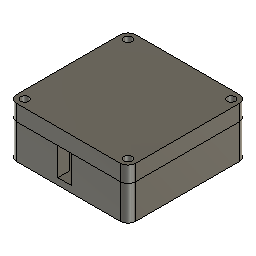
Wireless Charching Case (Autodesk Fusion 360 design; units mm, degrees)
Autodesk Fusion 360 part; units mm, degrees
sketch "Skizze1" plane through (0, 0, 0) normal (0, 0, 1) x (1, 0, 0)
  line L0 (15, -17.5) -> (-15, -17.5)
  line L1 (-17.5, -15) -> (-17.5, 15)
  line L2 (-15, 17.5) -> (15, 17.5)
  line L3 (17.5, 15) -> (17.5, -15)
  line L4 (17.5, -17.5) -> (-17.5, 17.5) construction
  line L5 (-17.5, -17.5) -> (17.5, 17.5) construction
  circle A0 centre (-15, 15) radius 1.5
  arc A1 (-15, 17.5) -> (-17.5, 15) centre (-15, 15) ccw
  arc A2 (-17.5, -15) -> (-15, -17.5) centre (-15, -15) ccw
  arc A3 (15, -17.5) -> (17.5, -15) centre (15, -15) ccw
  arc A4 (17.5, 15) -> (15, 17.5) centre (15, 15) ccw
  circle A5 centre (15, 15) radius 1.5
  circle A6 centre (-15, -15) radius 1.5
  circle A7 centre (15, -15) radius 1.5
  dimension "d1" = 35
  dimension "d2" = 35
  dimension "d3" = 3
  dimension "d4" = 2.5
  dimension "d5" = 2.5
  dimension "d8" = 30
  dimension "d9" = -30
  constraint horizontal L0
  constraint perpendicular L0 L1
  constraint parallel L0 L2
  constraint parallel L1 L3
  constraint coincident L4 origin
  constraint coincident L5 origin
  constraint coincident L4 A0.centre
  constraint coincident L4.end L2
  constraint coincident L4.end L1
  constraint tangent L2 A1
  constraint tangent L1 A1
  constraint coincident L5.start L1
  constraint coincident L5.start L0
  constraint tangent L1 A2
  constraint tangent L0 A2
  constraint equal A1 A2
  constraint coincident L4.start L0
  constraint coincident L4.start L3
  constraint tangent L0 A3
  constraint tangent L3 A3
  constraint equal A1 A3
  constraint coincident L5.end L3
  constraint coincident L5.end L2
  constraint tangent L3 A4
  constraint tangent L2 A4
  constraint equal A1 A4
  measures "d1" distance of L4.end L5.end
  measures "d2" distance of L5.start L4.end
  measures "d3" diameter of A0
  measures "d5" distance of L2 A0.centre
sketch "Skizze2" plane through (0, 0, 0) normal (0, 0, 1) x (1, 0, 0)
  line L0 (19.5, -22.5) -> (-19.5, -22.5)
  line L1 (-22.5, -19.5) -> (-22.5, 19.5)
  line L2 (-19.5, 22.5) -> (19.5, 22.5)
  line L3 (22.5, 19.5) -> (22.5, -19.5)
  line L4 (22.5, -22.5) -> (-22.5, 22.5) construction
  line L5 (-22.5, -22.5) -> (22.5, 22.5) construction
  arc A0 (-19.5, 22.5) -> (-22.5, 19.5) centre (-19.5, 19.5) ccw
  arc A1 (22.5, 19.5) -> (19.5, 22.5) centre (19.5, 19.5) ccw
  arc A2 (19.5, -22.5) -> (22.5, -19.5) centre (19.5, -19.5) ccw
  arc A3 (-22.5, -19.5) -> (-19.5, -22.5) centre (-19.5, -19.5) ccw
  line L6 (15, -18) -> (-15, -18)
  line L7 (-18, -15) -> (-18, 15)
  line L8 (-15, 18) -> (15, 18)
  line L9 (18, 15) -> (18, -15)
  line L10 (18, -18) -> (-18, 18) construction
  line L11 (-18, -18) -> (18, 18) construction
  arc A4 (-15, 18) -> (-18, 15) centre (-15, 15) ccw
  arc A5 (-18, -15) -> (-15, -18) centre (-15, -15) ccw
  arc A6 (15, -18) -> (18, -15) centre (15, -15) ccw
  arc A7 (18, 15) -> (15, 18) centre (15, 15) ccw
  circle A8 centre (-19.5, 19.5) radius 1.5
  circle A9 centre (19.5, 19.5) radius 1.5
  circle A10 centre (-19.5, -19.5) radius 1.5
  circle A11 centre (19.5, -19.5) radius 1.5
  line L12 (-4, -18) -> (1, -18)
  line L13 (1, -18) -> (1, -22.5)
  line L14 (1, -22.5) -> (-4, -22.5)
  line L15 (-4, -22.5) -> (-4, -18)
  dimension "d10" = 45
  dimension "d11" = 45
  dimension "d12" = 3
  dimension "d13" = 3
  dimension "d24" = 3
  dimension "d25" = 3
  dimension "d28" = 39
  dimension "d29" = -39
  dimension "d30" = 5
  dimension "d31" = 14
  constraint horizontal L0
  constraint perpendicular L0 L1
  constraint parallel L0 L2
  constraint parallel L1 L3
  constraint coincident L4 origin
  constraint coincident L5 origin
  constraint coincident L4.end L2
  constraint coincident L4.end L1
  constraint tangent L2 A0
  constraint tangent L1 A0
  constraint coincident L5.end L2
  constraint coincident L5.end L3
  constraint tangent L2 A1
  constraint tangent L3 A1
  constraint equal A0 A1
  constraint coincident L4.start L3
  constraint coincident L4.start L0
  constraint tangent L3 A2
  constraint tangent L0 A2
  constraint equal A0 A2
  constraint coincident L5.start L0
  constraint coincident L5.start L1
  constraint tangent L0 A3
  constraint tangent L1 A3
  constraint equal A0 A3
  constraint horizontal L6
  constraint perpendicular L6 L7
  constraint parallel L6 L8
  constraint parallel L7 L9
  constraint coincident L10 origin
  constraint coincident L11 origin
  constraint coincident L4 L10.start
  constraint coincident L10.end L8
  constraint coincident L10.end L7
  constraint tangent L8 A4
  constraint tangent L7 A4
  constraint coincident L11.start L7
  constraint coincident L11.start L6
  constraint tangent L7 A5
  constraint tangent L6 A5
  constraint equal A4 A5
  constraint coincident L10.start L6
  constraint coincident L10.start L9
  constraint tangent L6 A6
  constraint tangent L9 A6
  constraint equal A4 A6
  constraint coincident L11.end L9
  constraint coincident L11.end L8
  constraint tangent L9 A7
  constraint tangent L8 A7
  constraint equal A4 A7
  constraint coincident L4 A0.centre
  constraint horizontal L12
  constraint vertical L13
  constraint horizontal L14
  constraint vertical L15
  constraint coincident L6 L12.start
  measures "d10" distance of L4.end L5.end
  measures "d11" distance of L5.start L4.end
  measures "d12" radius of A0
  measures "d13" radius of A4
  measures "d24" diameter of A8
  measures "d25" distance of L2 A0.centre
  measures "d30" distance of L12.start L12.end
  measures "d31" distance of L7 L15
extrude "Extrusion1" add sketch "Skizze2" along normal blind 2.5 makes body 1
extrude "Extrusion2" add sketch "Skizze2" along normal blind 13 contours L0 L1 L2 L3 A0 A1 A2 A3 L6 L7 L8 L9 A4 A5 A6 A7 L13 L15 bodies 1
extrude "Extrusion4" cut sketch "Skizze1" along normal blind 2.5 contours A0 | A5 | A6 | A7 bodies 1
thread "Gewinde1" "ISO Metric profile 3.0 M3x0.5 M3x0.5 6H" major diameter 3.086 minor diameter 2.529 pitch 0.5 angle 60 resizes the face on face at (-13.5019, 14.9252, 1.6667) on face at (16.4981, 14.9252, 1.6667) on face at (-13.5019, -15.0748, 1.6667) on face at (16.4981, -15.0748, 1.6667) on bodies 1
sketch "Skizze3" plane through (0, 0, 13) normal (0, 0, 1) x (-1, 0, 0)
  circle A0 centre (19.5, -19.5) radius 1.5
  circle A1 centre (-19.5, -19.5) radius 1.5
  circle A2 centre (19.5, 19.5) radius 1.5
  circle A3 centre (-19.5, 19.5) radius 1.5
  arc A4 (22.5, 19.5) -> (19.5, 22.5) centre (19.5, 19.5) ccw
  line L0 (19.5, 22.5) -> (4, 22.5)
  line L1 (4, 22.5) -> (4, 18)
  line L2 (4, 18) -> (15, 18)
  arc A5 (18, 15) -> (15, 18) centre (15, 15) ccw
  line L3 (18, 15) -> (18, -15)
  arc A6 (15, -18) -> (18, -15) centre (15, -15) ccw
  line L4 (15, -18) -> (-15, -18)
  arc A7 (-18, -15) -> (-15, -18) centre (-15, -15) ccw
  line L5 (-18, -15) -> (-18, 15)
  arc A8 (-15, 18) -> (-18, 15) centre (-15, 15) ccw
  line L6 (-15, 18) -> (-1, 18)
  line L7 (-1, 18) -> (-1, 22.5)
  line L8 (-1, 22.5) -> (-19.5, 22.5)
  arc A9 (-19.5, 22.5) -> (-22.5, 19.5) centre (-19.5, 19.5) ccw
  line L9 (-22.5, 19.5) -> (-22.5, -19.5)
  arc A10 (-22.5, -19.5) -> (-19.5, -22.5) centre (-19.5, -19.5) ccw
  line L10 (-19.5, -22.5) -> (19.5, -22.5)
  arc A11 (19.5, -22.5) -> (22.5, -19.5) centre (19.5, -19.5) ccw
  line L11 (22.5, -19.5) -> (22.5, 19.5)
  line L12 (-19.5, 22.5) -> (19.5, 22.5)
  line L13 (22.5, 19.5) -> (22.5, -19.5)
  line L14 (19.5, -22.5) -> (-19.5, -22.5)
  line L15 (-22.5, -19.5) -> (-22.5, 19.5)
  line L16 (-22.5, 22.5) -> (22.5, -22.5) construction
  line L17 (22.5, 22.5) -> (-22.5, -22.5) construction
  arc A12 (19.5, -22.5) -> (22.5, -19.5) centre (19.5, -19.5) ccw
  arc A13 (22.5, 19.5) -> (19.5, 22.5) centre (19.5, 19.5) ccw
  arc A14 (-19.5, 22.5) -> (-22.5, 19.5) centre (-19.5, 19.5) ccw
  arc A15 (-22.5, -19.5) -> (-19.5, -22.5) centre (-19.5, -19.5) ccw
  dimension "d32" = 45
  dimension "d33" = 45
  dimension "d34" = 3
  constraint horizontal L12
  constraint perpendicular L12 L13
  constraint parallel L12 L14
  constraint parallel L13 L15
  constraint coincident L16 origin
  constraint coincident L17 origin
  constraint coincident L16.end L14
  constraint coincident L16.end L13
  constraint tangent L14 A12
  constraint tangent L13 A12
  constraint coincident L17.start L13
  constraint coincident L17.start L12
  constraint tangent L13 A13
  constraint tangent L12 A13
  constraint equal A12 A13
  constraint coincident L16.start L12
  constraint coincident L16.start L15
  constraint tangent L12 A14
  constraint tangent L15 A14
  constraint equal A12 A14
  constraint coincident L17.end L15
  constraint coincident L17.end L14
  constraint tangent L15 A15
  constraint tangent L14 A15
  constraint equal A12 A15
  measures "d32" distance of L16.end L17.end
  measures "d33" distance of L17.start L16.end
  measures "d34" radius of A12
extrude "Extrusion5" add sketch "Skizze3" along normal blind 6 separate body makes body 2
